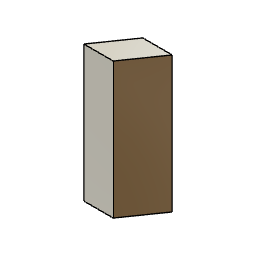
name_sign_support_right (Autodesk Fusion 360 design; units mm, degrees)
Autodesk Fusion 360 part; units mm, degrees
sketch "Name Sign Support" plane through (0, 0, 0) normal (1, 0, 0) x (0, 1, 0) in component "Name Sign Support (1)"
  line L0 (-0.0158, 97.2466) -> (23.9842, 87.4035)
  line L1 (23.9842, 142.8255) -> (-0.0158, 152.6686)
  line L2 (-0.0158, 152.6686) -> (-0.0158, 97.2466)
  line L3 (23.9842, 142.8255) -> (23.9842, 87.4035)
  dimension "d18" = 67.7
  dimension "d8" = 24
  dimension "d9" = 55.422
  constraint vertical L2
  constraint parallel L2 L3
  measures "d18" angle of L0 L3
  measures "d8" distance of L2 L3
  measures "d9" distance of L1.end L0.start
extrude "Extrude2" add sketch "Name Sign Support" along normal blind 12 in component "Name Sign Support (1)"
component "Name Sign Support Right" placed x (1, 0, 0) y (0, 1, 0) z (0, 0, 1) at (0, 0, 0)
component "Name Sign Support (1)" placed x (1, 0, 0) y (0, 1, 0) z (0, 0, 1) at (0, 0, 0) in component "Name Sign Support Right"
equation "d19 = pineThickness"
equation "pineThickness = 12 mm" comment "Thickness of the pine planks"
named bodies: "Name Sign Support"
